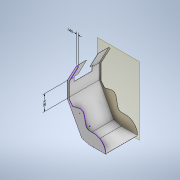
# Autodesk Inventor part: Seat3DSketch
Saved by Autodesk Inventor 2021 (Build 250183000, 183)
## iProperties
Created: 2020-10-04
Part Number: Seat3DSketch
Material: Generic
Document SubType Name: Modeling
Designer: PhotonUser
Density: 1 g/cm^3
Appearance: Default
Author: PhotonUser
Autodesk Inventor part; units mm, degrees
ref_plane "YZ Plane" through (0, 0, 0) normal (1, 0, 0) x (0, 1, 0)
ref_plane "XZ Plane" through (0, 0, 0) normal (0, 1, 0) x (-1, 0, 0)
sketch "Sketch1" plane through (0, 0, 0) normal (0, 0, 1) x (1, 0, 0)
  line L0 (0, 0) -> (-241.3, 0)
  line L1 (-352.8762, 28.575) -> (-241.3, 0)
  line L2 (-568.379, 431.8) -> (-352.8762, 28.575)
  arc A0 (-1.9317, 0) -> (-179.7317, 177.8) centre (-179.7317, 0) ccw
  arc A1 (-321.8515, 344.496) -> (-394.4455, 390.1126) centre (-380.6333, 331.522) ccw
  line L3 (-179.7317, 177.8) -> (-238.6526, 177.8)
  line L4 (-321.8515, 344.496) -> (-296.6352, 230.2477)
  arc A2 (-296.6352, 230.2477) -> (-238.6526, 177.8) centre (-238.6526, 236.0747) ccw
  line L5 (-490.4406, 367.4826) -> (-394.4455, 390.1126)
  line L6 (-568.379, 431.8) -> (-568.379, 660.4)
  line L7 (-542.979, 660.4) -> (-542.979, 431.8)
  line L8 (-542.979, 431.8) -> (-490.4406, 367.4826)
  line L9 (-431.7117, 914.4) -> (-568.379, 660.4)
  line L10 (-406.3016, 914.4) -> (-542.979, 660.4)
  line L11 (-406.3016, 914.4) -> (-431.7117, 914.4)
  constraints: 24 end point, 6 point on circle, 3 centre point, 3 horizontal, 3 point on line, 2 tangent, 1 vertical
sketch "Sketch4" plane through (0, 0, 0) normal (0, 0, 1) x (1, 0, 0)
  line L0 (-0.2535, 0) -> (-241.5535, 0)
  line L1 (-353.1324, 28.571) -> (-241.5535, 0)
  line L2 (-568.6352, 431.796) -> (-353.1324, 28.571)
  line L3 (-568.6352, 431.796) -> (-568.6352, 652.411)
  line L4 (-565.4602, 651.6325) -> (-565.4602, 432.585)
  line L5 (-431.9451, 914.3967) -> (-568.6352, 652.411)
  line L6 (-428.3639, 914.3967) -> (-565.4602, 651.6325)
  line L7 (-428.3639, 914.3967) -> (-431.9451, 914.3967)
  line L8 (-2.1852, 0) -> (-2.1852, 3.175)
  line L9 (-241.5535, 0) -> (-228.8535, 0)
  line L10 (-228.8535, 0) -> (-228.8535, 3.175)
  line L11 (-2.1852, 3.175) -> (-228.8535, 3.175)
  line L12 (-241.5535, 0) -> (-241.5535, 3.175)
  line L13 (-353.1324, 28.571) -> (-353.1324, 31.746)
  line L14 (-353.1324, 31.746) -> (-241.5535, 3.175)
  line L15 (-353.1324, 31.746) -> (-565.4602, 432.585)
  line L16 (-241.5535, 3.175) -> (-228.8535, 3.175)
  line L17 (-565.4602, 432.585) -> (-568.2578, 431.0898)
  line L18 (-565.4602, 651.6325) -> (-568.6352, 652.411)
  point P0 (0, 0)
  dimension "d63" = 3.175
  dimension "d64" = 12.7
  dimension "d65" = 3.175
  dimension "d66" = 3.175
  dimension "d68" = 3.175
  dimension "d90" = 3.175
  dimension "d92" = 3.175
  dimension "d93" = 3.175
  dimension "d96" = 0
  dimension "d97" = 0
  constraints: 38 end point, 4 point on line, 3 vertical, 2 horizontal, 1 collinear, 1 perpendicular
  measures "d63" distance of L8.start L8.end
  measures "d64" distance of L0.end L9.end
  measures "d65" distance of L9.end L10.end
  measures "d66" distance of L0.end L12.end
  measures "d68" distance of L1.start L13.end
  measures "d90" distance from line of L15 L2.start
  measures "d92" distance between parallel lines of L3 L4
  measures "d93" distance from line of L6.start L5
  measures "d96" angle of L6 L5
  measures "d97" distance of L7.end L5.start
extrude "Extrusion1" add sketch "Sketch4" against normal blind 469.9
extrude "Extrusion2" add sketch "Sketch1" along normal blind 3.175
ref_plane "Work Plane3" through (0, 0, -469.9) normal (0, 0, 1) x (1, 0, 0)
sketch "Sketch5" plane through (0, 0, 0) normal (0, 0, 1) x (1, 0, 0)
  line L0 (0, 0) -> (-241.3, 0)
  line L1 (-352.8762, 28.575) -> (-241.3, 0)
  line L2 (-568.379, 431.8) -> (-352.8762, 28.575)
  arc A0 (-1.9317, 0) -> (-179.7317, 177.8) centre (-179.7317, 0) ccw
  arc A1 (-321.8515, 344.496) -> (-394.4455, 390.1126) centre (-380.6333, 331.522) ccw
  line L3 (-179.7317, 177.8) -> (-238.6526, 177.8)
  line L4 (-321.8515, 344.496) -> (-296.6352, 230.2477)
  arc A2 (-296.6352, 230.2477) -> (-238.6526, 177.8) centre (-238.6526, 236.0747) ccw
  line L5 (-490.4406, 367.4826) -> (-394.4455, 390.1126)
  line L6 (-568.379, 431.8) -> (-568.379, 660.4)
  line L7 (-542.979, 660.4) -> (-542.979, 431.8)
  line L8 (-542.979, 431.8) -> (-490.4406, 367.4826)
  line L9 (-431.7117, 914.4) -> (-568.379, 660.4)
  line L10 (-406.3016, 914.4) -> (-542.979, 660.4)
  line L11 (-406.3016, 914.4) -> (-431.7117, 914.4)
  constraints: 24 end point, 6 point on circle, 3 centre point, 3 horizontal, 3 point on line, 2 tangent, 1 vertical
sketch "Sketch6" plane through (0, 0, -469.9) normal (0, 0, 1) x (1, 0, 0)
  point P0 (0, 0)
sketch "Sketch7" plane through (0, 0, -469.9) normal (0, 0, 1) x (1, 0, 0)
  line L0 (0, 0) -> (-241.3, 0)
  line L1 (-352.8762, 28.575) -> (-241.3, 0)
  line L2 (-568.379, 431.8) -> (-352.8762, 28.575)
  arc A0 (-1.9317, 0) -> (-179.7317, 177.8) centre (-179.7317, 0) ccw
  arc A1 (-321.8515, 344.496) -> (-394.4455, 390.1126) centre (-380.6333, 331.522) ccw
  line L3 (-179.7317, 177.8) -> (-238.6526, 177.8)
  line L4 (-321.8515, 344.496) -> (-296.6352, 230.2477)
  arc A2 (-296.6352, 230.2477) -> (-238.6526, 177.8) centre (-238.6526, 236.0747) ccw
  line L5 (-490.4406, 367.4826) -> (-394.4455, 390.1126)
  line L6 (-568.379, 431.8) -> (-568.379, 660.4)
  line L7 (-542.979, 660.4) -> (-542.979, 431.8)
  line L8 (-542.979, 431.8) -> (-490.4406, 367.4826)
  line L9 (-431.7117, 914.4) -> (-568.379, 660.4)
  line L10 (-406.3016, 914.4) -> (-542.979, 660.4)
  line L11 (-406.3016, 914.4) -> (-431.7117, 914.4)
  constraints: 24 end point, 6 point on circle, 3 centre point, 3 horizontal, 3 point on line, 2 tangent, 1 vertical
extrude "Extrusion3" add sketch "Sketch7" against normal blind 3.175
sketch "Sketch8" plane through (0, 0, 0) normal (1, 0, 0) x (0, 1, 0)
  line L0 (0, 0) -> (0, -228.6)
  line L1 (0, -473.075) -> (0, 3.175) projected
  line L2 (0, -228.6) -> (596.9, -228.6)
  line L3 (651.6325, -473.075) -> (651.6325, 3.175) projected
  line L4 (596.9, -228.6) -> (596.9, -95.25)
  line L5 (432.585, 0) -> (432.585, -469.9) projected
  line L6 (596.9, -228.6) -> (596.9, -361.95)
  line L7 (596.9, -361.95) -> (1104.9, -361.95)
  line L8 (1104.9, -361.95) -> (1104.9, -95.25)
  line L9 (1104.9, -95.25) -> (596.9, -95.25)
  line L10 (596.9, -95.25) -> (651.6325, -95.25)
  line L11 (651.6325, -95.25) -> (677.0325, -95.25)
  line L12 (677.0325, -95.25) -> (677.0325, -142.875)
  line L13 (677.0325, -142.875) -> (1104.9, -142.875)
  line L14 (651.6325, -361.95) -> (685.8, -361.95)
  line L15 (685.8, -361.95) -> (685.8, -314.325)
  line L16 (685.8, -314.325) -> (1104.9, -314.325)
  point P0 (660.4, -473.075)
  point P1 (660.4, 3.175)
  point P2 (431.8, 0)
  point P3 (431.8, -469.9)
  point P4 (432.585, -469.9)
  dimension "d77" = 228.6
  dimension "d78" = 596.9
  dimension "d80" = 133.35
  dimension "d81" = 133.35
  dimension "d82" = 508
  dimension "d83" = 266.7
  dimension "d84" = 25.4
  dimension "d85" = 47.625
  dimension "d86" = 47.625
  constraints: 28 end point, 7 point on line, 5 perpendicular, 3 vertical, 1 horizontal, 4 other
  measures "d77" distance of L0.start L0.end
  measures "d78" distance of L0.end L2.end
  measures "d80" distance of L2.end L4.end
  measures "d81" distance of L2.end L6.end
  measures "d82" distance of L6.end L7.end
  measures "d83" distance of L7.end L8.end
  measures "d84" distance of L10.end L11.end
  measures "d85" distance of L11.end L12.end
  measures "d86" distance of L14.end L15.end
extrude "Extrusion4" cut sketch "Sketch8" against normal blind 914.4 contours L7 L6 L4 L9 L3 | L3 L9 L12 L13 L8 L16 L15 L7
equation "\"SeatBottomDepth\" = 241.3"
equation "\"SeatFrontBottomWidth\" = 469.9"
equation "\"SeatFrontSidesWidth\" = 520.7"
equation "\"SeatBackInnerWidth\" = 304.8"
equation "\"SeatBackOuterWidth\" = 482.6"
equation "\"SeatBackLength\" = 457.2"
body "Solid1"
